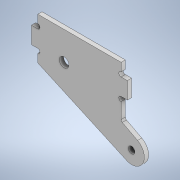
# Autodesk Inventor part: 付け根_メインフレーム
Saved by Autodesk Inventor 2020 (Build 240168000, 168)
## iProperties
Created: 2021-09-05
Part Number: 付け根_メインフレーム
Material: Generic
Document SubType Name: Modeling
Designer: masato
Density: 1 g/cm^3
Appearance: Default
Mass: 2.49664 g
Surface Area: 28.7716 cm^2
Volume: 2.49664 cm^3
Author: masato
Autodesk Inventor part; units mm, degrees
ref_plane "YZ Plane" through (0, 0, 0) normal (1, 0, 0) x (0, 1, 0)
ref_plane "XZ Plane" through (0, 0, 0) normal (0, 1, 0) x (-1, 0, 0)
ref_plane "XY Plane" through (0, 0, 0) normal (0, 0, 1) x (1, 0, 0)
sketch "スケッチ1" plane through (0, 0, 0) normal (0, 0, 1) x (1, 0, 0)
  line L0 (-19.75, 25.75) -> (19.75, 25.75) construction
  line L1 (19.75, 25.75) -> (19.75, -25.75) construction
  line L2 (19.75, -25.75) -> (-19.75, -25.75) construction
  line L3 (-19.75, -25.75) -> (-19.75, 25.75) construction
  line L4 (-19.75, 25.75) -> (19.75, -25.75) construction
  line L5 (19.75, 25.75) -> (-19.75, -25.75) construction
  circle A0 centre (24.75, -24.25) radius 1.55
  circle A1 centre (-7.25, -4.25) radius 2.25
  line L6 (0, 25.75) -> (0, -25.75) construction
  line L7 (-19.75, 3.25) -> (-22.75, 3.25)
  line L8 (-22.75, 3.25) -> (-22.75, -4.75)
  arc A2 (-19.75, 3.25) -> (-19.75, 5.35) centre (-19.75, 4.3) ccw
  line L9 (-22.75, -0.75) -> (-19.75, -0.75) construction
  line L10 (-19.75, -4.75) -> (-22.75, -4.75)
  arc A3 (-19.75, -6.85) -> (-19.75, -4.75) centre (-19.75, -5.8) ccw
  line L11 (-19.75, 5.35) -> (-19.75, 9.25)
  line L12 (-19.75, 9.25) -> (19.75, 9.25)
  line L13 (22.75, 3.25) -> (22.75, -4.75)
  arc A4 (19.75, 5.35) -> (19.75, 3.25) centre (19.75, 4.3) ccw
  line L14 (19.75, -4.75) -> (22.75, -4.75)
  arc A5 (19.75, -4.75) -> (19.75, -6.85) centre (19.75, -5.8) ccw
  line L15 (19.75, 5.35) -> (19.75, 9.25)
  line L16 (19.75, 3.25) -> (22.75, 3.25)
  arc A6 (22.2819, -29.7189) -> (27.5381, -18.9372) centre (24.75, -24.25) ccw
  line L17 (-19.75, -6.85) -> (-19.75, -10.75)
  line L18 (-19.75, -10.75) -> (22.2819, -29.7189)
  line L19 (19.75, -6.85) -> (19.75, -14.85)
  line L20 (19.75, -14.85) -> (27.5381, -18.9372)
  point P0 (0, 0)
  dimension "d0" = 39.5
  dimension "d1" = 51.5
  dimension "d2" = 3.1
  dimension "d3" = 4.5
  dimension "d4" = 32
  dimension "d5" = 20
  dimension "d6" = 3
  dimension "d7" = 1.05
  dimension "d8" = 8
  dimension "d9" = 26.5
  dimension "d11" = 30
  dimension "d12" = 12.5
  dimension "d13" = 6
  dimension "d14" = 12
  dimension "d17" = 8
  constraints: 42 end point, 12 symmetric about line, 10 point on circle, 7 centre point, 7 point on line, 5 midpoint, 4 perpendicular, 2 horizontal, 2 parallel, 2 tangent, 1 coincident, 3 other
  measures "d0" distance of L1.end L2.end
  measures "d1" distance of L0.end L1.end
  measures "d2" diameter of A0
  measures "d3" diameter of A1
  measures "d4" horizontal distance of A0.centre A1.centre
  measures "d5" vertical distance of A0.centre A1.centre
  measures "d6" distance of L7.start L7.end
  measures "d7" radius of A2
  measures "d8" distance of L7.end L8.end
  measures "d9" vertical distance of L0.start L9.start
  measures "d11" vertical distance of L0.start A1.centre
  measures "d12" horizontal distance of A1.centre L0.start
  measures "d13" vertical distance of L7.end L11.end
  measures "d14" diameter of A6
  measures "d17" distance of L19.start L19.end
extrude "押し出し1" add sketch "スケッチ1" along normal blind 2
fillet "フィレット1" radius 1 1 edges at (19.75, -14.85, 1)
